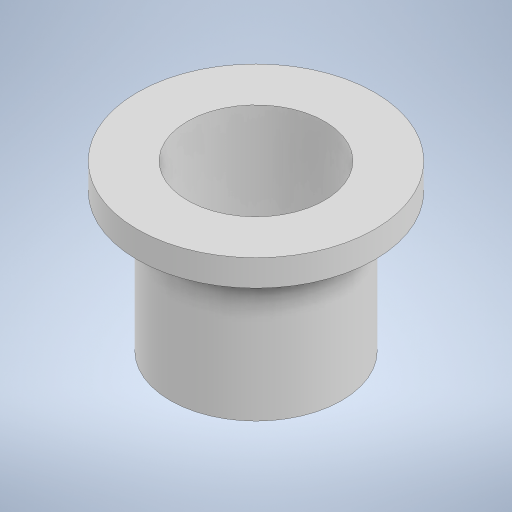
# Autodesk Inventor part: Pieza LED
Saved by Autodesk Inventor 2024 (Build 280153000, 153)
## iProperties
Created: 2023-06-24
Part Number: Pieza LED
Material: Genérico
Document SubType Name: Modeling
Designer: sergi
Density: 1 g/cm^3
Appearance: Valor por defecto
Author: sergi
Autodesk Inventor part; units mm, degrees
ref_plane "YZ Plane" through (0, 0, 0) normal (1, 0, 0) x (0, 1, 0)
ref_plane "XZ Plane" through (0, 0, 0) normal (0, 1, 0) x (-1, 0, 0)
ref_plane "XY Plane" through (0, 0, 0) normal (0, 0, 1) x (1, 0, 0)
sketch "Boceto1" plane through (0, 0, 0) normal (0, 1, 0) x (-1, 0, 0)
  circle A0 centre (0, 0) radius 2.6
  circle A1 centre (0, 0) radius 3.25
  dimension "d0" = 5.2
  dimension "d1" = 6.5
  constraints: 2 centre point, 2 coincident
  measures "d0" diameter of A0
  measures "d1" diameter of A1
extrude "Extrusión1" add sketch "Boceto1" along normal blind 6.25
sketch "Boceto2" plane through (0, 6.25, 0) normal (0, 1, 0) x (1, 0, 0)
  circle A0 centre (0, 0) radius 4.5
  circle A1 centre (0, 0) radius 3.25 projected
  circle A2 centre (0, 0) radius 3.25 projected
  circle A3 centre (0, 0) radius 2.6 projected
  dimension "d4" = 9
  constraints: 1 centre point, 1 coincident
  measures "d4" diameter of A0
extrude "Extrusión2" add sketch "Boceto2" against normal blind 1 contours A0
